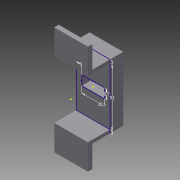
# Autodesk Inventor part: servo halter
Saved by Autodesk Inventor 2015 (Build 190159000, 159)
## iProperties
Created: 2016-09-20
Part Number: servo halter
Material: Generic
Document SubType Name: Modeling
Designer: moritz
Density: 1 g/cm^3
Appearance: Default
Author: moritz
Autodesk Inventor part; units mm, degrees
ref_plane "YZ Plane" through (0, 0, 0) normal (1, 0, 0) x (0, 1, 0)
ref_plane "XZ Plane" through (0, 0, 0) normal (0, 1, 0) x (-1, 0, 0)
ref_plane "XY Plane" through (0, 0, 0) normal (0, 0, 1) x (1, 0, 0)
sketch "Sketch1" plane through (0, 0, 0) normal (0, 1, 0) x (-1, 0, 0)
  line L0 (10.25, 4.35) -> (-10.25, 4.35)
  line L1 (-10.25, 4.35) -> (-10.25, -4.35)
  line L2 (-10.25, -4.35) -> (10.25, -4.35)
  line L3 (10.25, -4.35) -> (10.25, 4.35)
  line L4 (15.25, 26) -> (-15.25, 26)
  line L5 (-15.25, 26) -> (-15.25, -26)
  line L6 (-15.25, -26) -> (15.25, -26)
  line L7 (15.25, -26) -> (15.25, 26)
  line L8 (15.25, 26) -> (-15.25, 26)
  line L9 (-15.25, 26) -> (-15.25, 29)
  line L10 (-15.25, 29) -> (15.25, 29)
  line L11 (15.25, 29) -> (15.25, 26)
  line L12 (15.25, -26) -> (-15.25, -26)
  line L13 (-15.25, -26) -> (-15.25, -29)
  line L14 (-15.25, -29) -> (15.25, -29)
  line L15 (15.25, -29) -> (15.25, -26)
  point P0 (0, 0)
  point P1 (0, 4.35)
  point P2 (10.25, 0)
  point P3 (0, 26)
  point P4 (15.25, 0)
  dimension "d0" = 8.7
  dimension "d1" = 20.5
  dimension "d2" = 52
  dimension "d3" = 5
  dimension "d4" = 3
  dimension "d5" = 3
  constraints: 32 end point, 8 parallel, 4 horizontal, 4 midpoint, 4 perpendicular, 2 horizontal alignment, 2 point on line, 2 vertical alignment
  measures "d0" distance of L1.end L0.end
  measures "d1" distance between parallel lines of L1 L3
  measures "d2" distance of L5.end L4.end
  measures "d3" distance between parallel lines of L7 L3
  measures "d4" distance of L8.end L9.end
  measures "d5" distance of L13.end L12.end
extrude "Extrusion1" add sketch "Sketch1" along normal blind 12
extrude "Extrusion2" add sketch "Sketch1" against normal blind 20 contours L4 L9 L10 L11 | L15 L14 L13 L6
sketch "Sketch2" plane through (0, -20, 0) normal (0, -1, 0) x (1, 0, 0)
  point P0 (0, 0)
sketch "Sketch3" plane through (-15.25, 12, 29) normal (0, 0, 1) x (1, 0, 0)
  line L0 (30.5, -32) -> (30.5, 0) projected
  line L1 (0, 0) -> (30.5, 0) projected
  line L2 (0, -32) -> (0, 0) projected
  line L3 (30.5, -32) -> (0, -32) projected
  line L4 (0, -32) -> (0, 0) projected
  line L5 (30.5, -32) -> (0, -32)
  line L6 (0, -32) -> (0, -28)
  line L7 (0, -28) -> (30.5, -28)
  line L8 (30.5, -28) -> (30.5, -32)
  point P0 (15.25, -12)
  dimension "d10" = 4
  constraints: 8 end point, 2 parallel, 1 horizontal, 1 perpendicular, 1 point on line
  measures "d10" distance of L5.end L6.end
sketch "Sketch4" plane through (15.25, 12, -29) normal (0, 0, -1) x (-1, 0, 0)
  line L0 (30.5, -32) -> (30.5, 0) projected
  line L1 (0, 0) -> (30.5, 0) projected
  line L2 (0, -32) -> (0, 0) projected
  line L3 (30.5, -32) -> (0, -32) projected
  line L4 (30.5, -32) -> (30.5, 0) projected
  line L5 (0, -32) -> (30.5, -32)
  line L6 (30.5, -32) -> (30.5, -28)
  line L7 (30.5, -28) -> (0, -28)
  line L8 (0, -28) -> (0, -32)
  point P0 (15.25, -12)
  dimension "d11" = 4
  constraints: 8 end point, 2 parallel, 1 horizontal, 1 perpendicular, 1 point on line
  measures "d11" distance of L6.end L5.end
extrude "Extrusion3" add sketch "Sketch4" along normal blind 20 contours L3 L2 L7 L0
extrude "Extrusion4" add sketch "Sketch3" along normal blind 20 contours L3 L2 L7 L0
shell "Shell1" thickness 3 removed faces 1 at (-3.4167, 12, -20.7833)
chamfer "Chamfer1" distance 9 angle 45 2 edges at (-12.25, 3, -16.675) (-12.25, 3, 16.675)
body "Solid1"
